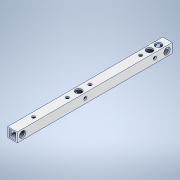
# Autodesk Inventor part: 上下直動9x9_3
Saved by Autodesk Inventor 2020.3 (Build 243373000, 373)
## iProperties
Created: 2020-07-05
Part Number: 上下直動9x9_3
Material: アルミニウム 6061
Document SubType Name: Modeling
Designer: totot
Density: 2.7 g/cm^3
Appearance: アルミニウム - フラット
Mass: 14.2187 g
Surface Area: 90.7803 cm^2
Volume: 5.26618 cm^3
Author: totot
Autodesk Inventor part; units mm, degrees
ref_plane "YZ Plane" through (0, 0, 0) normal (1, 0, 0) x (0, 1, 0)
ref_plane "XZ Plane" through (0, 0, 0) normal (0, 1, 0) x (-1, 0, 0)
ref_plane "XY Plane" through (0, 0, 0) normal (0, 0, 1) x (1, 0, 0)
sketch "スケッチ1" plane through (0, 0, 0) normal (0, 0, 1) x (1, 0, 0)
  line L0 (0, 0) -> (9, 0)
  line L1 (9, 0) -> (9, -9)
  line L2 (9, -9) -> (0, -9)
  line L3 (0, -9) -> (0, 0)
  line L4 (1.2, -1.2) -> (7.8, -1.2)
  line L5 (7.8, -1.2) -> (7.8, -7.8)
  line L6 (7.8, -7.8) -> (1.2, -7.8)
  line L7 (1.2, -7.8) -> (1.2, -1.2)
  dimension "d0" = 9
  dimension "d1" = 9
  dimension "d2" = 6.6
  dimension "d3" = 6.6
  dimension "d4" = 1.2
  dimension "d5" = 1.2
  constraints: 16 end point, 4 parallel, 2 horizontal, 2 perpendicular
  measures "d0" distance of L1.end L2.end
  measures "d1" distance of L0.end L1.end
  measures "d2" distance of L5.end L6.end
  measures "d3" distance of L4.end L5.end
  measures "d4" distance between parallel lines of L3 L7
  measures "d5" distance between parallel lines of L4 L0
extrude "押し出し1" add sketch "スケッチ1" along normal blind 75
sketch "スケッチ2" plane through (9, -9, 0) normal (1, 0, 0) x (0, 0, -1)
  line L0 (0, 9) -> (-75, 9) projected
  line L1 (0, 0) -> (0, 9) projected
  line L2 (-75, 0) -> (-75, 9) projected
  point P0 (-70.5, 4.5)
  point P1 (-4.5, 4.5)
  dimension "d8" = 4.5
  dimension "d9" = 4.5
  dimension "d10" = 4.5
  dimension "d11" = 4.5
  measures "d8" distance from line of point (-70.5, 4.5) L0
  measures "d9" distance from line of point (-4.5, 4.5) L0
  measures "d10" distance from line of point (-4.5, 4.5) L1
  measures "d11" distance from line of L2 point (-70.5, 4.5)
hole "穴1" at (9, -4.5, 70.5) at (9, -4.5, 4.5) direction (-1, 0, 0) diameter 3 end through all
sketch "スケッチ3" plane through (0, 0, 0) normal (0, 1, 0) x (1, 0, 0)
  line L0 (0, 0) -> (0, -75) projected
  line L1 (9, 0) -> (0, 0) projected
  line L2 (9, -75) -> (0, -75) projected
  point P0 (4.5, -61.5)
  point P1 (4.5, -13.5)
  dimension "d19" = 4.5
  dimension "d20" = 4.5
  dimension "d21" = 13.5
  dimension "d22" = 13.5
  measures "d19" distance from line of point (4.5, -61.5) L0
  measures "d20" distance from line of point (4.5, -13.5) L0
  measures "d21" distance from line of point (4.5, -13.5) L1
  measures "d22" distance from line of point (4.5, -61.5) L2
hole "穴2" at (4.5, 0, 61.5) at (4.5, 0, 13.5) direction (0, -1, 0) diameter 3 end through all
sketch "スケッチ6" plane through (0, 0, 75) normal (0, 0, 1) x (1, 0, 0)
  line L0 (0, -9) -> (9, -9) projected
  line L1 (0, 0) -> (9, 0)
  line L2 (9, 0) -> (9, -9)
  line L3 (9, -9) -> (0, -9)
  line L4 (0, -9) -> (0, 0)
  line L5 (1.2, -1.2) -> (7.8, -1.2) projected
  line L6 (7.8, -1.2) -> (7.8, -7.8) projected
  line L7 (1.2, -1.2) -> (7.8, -1.2)
  line L8 (7.8, -1.2) -> (7.8, -7.8)
  line L9 (7.8, -7.8) -> (1.2, -7.8)
  line L10 (1.2, -7.8) -> (1.2, -1.2)
  constraints: 16 end point, 4 parallel, 2 horizontal, 2 perpendicular
extrude "押し出し3" add sketch "スケッチ6" along normal blind 60
sketch "スケッチ7" plane through (9, -9, 0) normal (1, 0, 0) x (0, 0, -1)
  line L0 (-135, 0) -> (-135, 9) projected
  line L1 (0, 9) -> (-135, 9) projected
  point P0 (-130, 4.5)
  dimension "d43" = 5
  dimension "d44" = 4.5
  measures "d43" distance from line of point (-130, 4.5) L0
  measures "d44" distance from line of point (-130, 4.5) L1
hole "穴4" at (9, -4.5, 130) direction (-1, 0, 0) diameter 6 end through all
sketch "スケッチ8" plane through (0, 0, 0) normal (0, 0, -1) x (-1, 0, 0)
  line L0 (-9, -9) -> (-9, 0) projected
  line L1 (0, 0) -> (-9, 0)
  line L2 (-9, 0) -> (-9, -9)
  line L3 (-9, -9) -> (0, -9)
  line L4 (0, -9) -> (0, 0)
  line L5 (-7.8, -7.8) -> (-1.2, -7.8) projected
  line L6 (-7.8, -7.8) -> (-1.2, -7.8)
  line L7 (-1.2, -7.8) -> (-1.2, -1.2)
  line L8 (-1.2, -1.2) -> (-7.8, -1.2)
  line L9 (-7.8, -1.2) -> (-7.8, -7.8)
  constraints: 16 end point, 4 parallel, 2 horizontal, 2 perpendicular
extrude "押し出し4" add sketch "スケッチ8" along normal blind 12
sketch "スケッチ9" plane through (0, -9, 135) normal (-1, 0, 0) x (0, 0, 1)
  line L0 (-147, 0) -> (-147, 9) projected
  line L1 (0, 0) -> (-147, 0) projected
  point P0 (-135, 9)
  point P1 (-142, 4.5)
  dimension "d54" = 5
  dimension "d55" = 4.5
  measures "d54" distance from line of point (-142, 4.5) L0
  measures "d55" distance from line of point (-142, 4.5) L1
hole "穴5" at (0, -4.5, -7) direction (1, 0, 0) diameter 6 end through all
sketch "スケッチ10" plane through (0, -9, 135) normal (0, -1, 0) x (1, 0, 0)
  line L0 (0, 0) -> (9, 0) projected
  line L1 (0, 0) -> (0, -147) projected
  point P0 (0, -135)
  point P1 (4.5, -52)
  point P2 (4.5, -20)
  dimension "d63" = 20
  dimension "d64" = 32
  dimension "d65" = 4.5
  dimension "d66" = 4.5
  measures "d63" distance from line of point (4.5, -20) L0
  measures "d64" distance of point (4.5, -20) point (4.5, -52)
  measures "d65" distance from line of L1 point (4.5, -20)
  measures "d66" distance from line of point (4.5, -52) L1
hole "穴6" at (4.5, -9, 83) at (4.5, -9, 115) direction (0, 1, 0) diameter 3 end through all
sketch "スケッチ11" plane through (0, -9, 135) normal (-1, 0, 0) x (0, 0, 1)
  point P0 (-135, 9)
sketch "スケッチ12" plane through (0, 0, 135) normal (0, 1, 0) x (1, 0, 0)
  line L0 (0, 147) -> (0, 0) projected
  line L1 (0, 147) -> (9, 147) projected
  circle A0 centre (4.5, 121.5) radius 1.5 projected
  point P0 (0, 135)
  point P1 (4.5, 138.5)
  point P2 (4.5, 130)
  dimension "d74" = 4.5
  dimension "d75" = 25.5
  dimension "d76" = 8.5
  dimension "d77" = 8.5
  dimension "d78" = 4.5
  measures "d74" distance from line of L0 point (4.5, 138.5)
  measures "d75" distance from line of L1 A0.centre
  measures "d76" distance from line of point (4.5, 138.5) L1
  measures "d77" distance of point (4.5, 130) point (4.5, 138.5)
  measures "d78" distance from line of point (4.5, 130) L0
hole "穴7" at (4.5, 0, 5) at (4.5, 0, -3.5) direction (0, -1, 0) diameter 6 end through all
sketch "スケッチ13" plane through (0, 0, 135) normal (0, 1, 0) x (1, 0, 0)
  circle A0 centre (4.5, 52) radius 1.5 projected
  circle A1 centre (4.5, 73.5) radius 1.5 projected
  line L0 (0, 147) -> (0, 0) projected
  point P0 (0, 135)
  point P1 (4.5, 62.75)
  dimension "d86" = 21.5
  dimension "d87" = 10.75
  dimension "d88" = 4.5
  measures "d86" distance of A0.centre A1.centre
  measures "d87" distance of point (4.5, 62.75) A1.centre
  measures "d88" distance from line of point (4.5, 62.75) L0
hole "穴8" at (4.5, 0, 72.25) direction (0, -1, 0) diameter 6 end through all
equation "\"d10\" = d9"
equation "\"d22\" = d21"
equation "\"d76\" = 0.333333 * d75"
equation "\"d77\" = d76"
equation "\"d87\" = 0.5 * d86"
